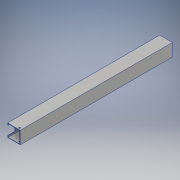
# Autodesk Inventor part: TelescopeOuter
Saved by Autodesk Inventor 2018.3 (Build 223284000, 284)
## iProperties
Created: 2020-01-18
Part Number: TelescopeOuter
Material: Aluminum 6061
Document SubType Name: Modeling
Designer: Cooper
Density: 2.7 g/cm^3
Appearance: Aluminum - Flat
Mass: 387.063 g
Surface Area: 1812.88 cm^2
Volume: 143.357 cm^3
Author: Cooper
Autodesk Inventor part; units mm, degrees
ref_plane "YZ Plane" through (0, 0, 0) normal (1, 0, 0) x (0, 1, 0)
ref_plane "XZ Plane" through (0, 0, 0) normal (0, 1, 0) x (-1, 0, 0)
ref_plane "XY Plane" through (0, 0, 0) normal (0, 0, 1) x (1, 0, 0)
sketch "Sketch1" plane through (0, 0, 0) normal (0, 0, 1) x (1, 0, 0)
  line L0 (0, 0) -> (44.45, 0)
  line L1 (44.45, 0) -> (44.45, 44.45)
  line L2 (44.45, 44.45) -> (0, 44.45)
  line L3 (0, 44.45) -> (0, 0)
  line L4 (1.5875, 42.8625) -> (42.8625, 42.8625)
  line L5 (42.8625, 42.8625) -> (42.8625, 1.5875)
  line L6 (42.8625, 1.5875) -> (1.5875, 1.5875)
  line L7 (1.5875, 1.5875) -> (1.5875, 42.8625)
  dimension "d0" = 44.45
  dimension "d1" = 44.45
  dimension "d2" = 1.5875
  constraints: 16 end point, 4 parallel, 2 perpendicular, 1 horizontal, 3 other
  measures "d0" distance of L2.end L0.start
  measures "d1" distance of L0.start L0.end
  measures "d2" distance between parallel lines of L2 L4
extrude "Extrusion1" add sketch "Sketch1" along normal blind 533.4
sketch "Sketch2" plane through (44.45, 0, 0) normal (1, 0, 0) x (0, 0, -1)
  line L0 (0, 22.225) -> (-12.7, 22.225) construction
  line L1 (0, 12.7) -> (-12.7, 12.7)
  line L2 (-12.7, 31.75) -> (0, 31.75)
  arc A0 (0, 12.7) -> (0, 31.75) centre (0, 22.225) ccw
  arc A1 (-12.7, 31.75) -> (-12.7, 12.7) centre (-12.7, 22.225) ccw
  line L3 (0, 0) -> (0, 44.45) projected
  line L4 (0, 44.45) -> (-533.4, 44.45) projected
  point P0 (-6.35, 22.225)
  dimension "d5" = 0
  dimension "d7" = 19.05
  dimension "d20" = 12.7
  dimension "d21" = 22.225
  constraints: 8 end point, 4 point on circle, 4 tangent, 2 centre point, 1 horizontal, 1 midpoint, 1 parallel, 1 other
  measures "d7" distance between parallel lines of L1 L2
  measures "d20" distance of L1.start L1.end
  measures "d21" distance from line of L4 point (-6.35, 22.225)
extrude "Extrusion2" cut sketch "Sketch2" against normal blind 127
sketch "Sketch6" plane through (44.45, 0, 533.4) normal (1, 0, 0) x (0, 0, -1)
  line L0 (533.4, 42.8625) -> (533.4, 31.75) projected
  arc A0 (520.7, 31.75) -> (520.7, 12.7) centre (520.7, 22.225) ccw projected
  line L1 (533.4, 31.75) -> (520.7, 31.75)
  arc A1 (520.7, 31.75) -> (520.7, 12.7) centre (520.7, 22.225) ccw
  line L2 (533.4, 12.7) -> (520.7, 12.7) projected
  line L3 (520.7, 12.7) -> (533.4, 12.7)
  line L4 (533.4, 12.7) -> (533.4, 31.75)
  point P0 (533.4, 0)
  constraints: 6 end point, 2 horizontal, 2 point on circle, 2 tangent, 1 centre point, 1 perpendicular
extrude "Extrusion3" add sketch "Sketch6" against normal blind 1.5875
sketch "Sketch7" plane through (0, 0, 533.4) normal (-1, 0, 0) x (0, 0, 1)
  line L0 (0, 0) -> (0, 44.45) projected
  line L1 (0, 38.1) -> (-25.4, 38.1)
  line L2 (-25.4, 38.1) -> (-25.4, 6.35)
  line L3 (-25.4, 6.35) -> (0, 6.35)
  line L4 (0, 6.35) -> (0, 38.1)
  line L5 (-39.9502, 6.35) -> (-39.9502, 38.1)
  line L6 (-533.4, 31.75) -> (-520.7, 31.75) projected
  arc A0 (-520.7, 12.7) -> (-520.7, 31.75) centre (-520.7, 22.225) ccw projected
  line L7 (-520.7, 12.7) -> (-533.4, 12.7) projected
  line L8 (-533.4, 12.7) -> (-533.4, 0) projected
  line L9 (-533.4, 0) -> (0, 0) projected
  line L10 (0, 44.45) -> (0, 0) projected
  line L11 (-533.4, 44.45) -> (0, 44.45) projected
  line L12 (-533.4, 44.45) -> (-533.4, 31.75) projected
  dimension "d24" = 25.4
  dimension "d25" = 31.75
  dimension "d26" = 6.35
  dimension "d27" = 6.35
  constraints: 10 end point, 2 parallel, 1 horizontal, 1 perpendicular, 1 point on line, 1 vertical, 2 other
  measures "d24" distance of L1.start L1.end
  measures "d25" distance of L1.end L2.end
  measures "d26" distance between parallel lines of L1 L11
  measures "d27" distance between parallel lines of L9 L3
extrude "Extrusion4" cut sketch "Sketch7" against normal blind 1.5875 contours L3 L2 L1 L0
sketch "Sketch8" plane through (0, 0, 0) normal (0, -1, 0) x (1, 0, 0)
  line L0 (44.45, 0) -> (44.45, 533.4) projected
  line L1 (0, 533.4) -> (44.45, 533.4) projected
  point P0 (0, 0)
  point P1 (35.7188, 527.05)
  dimension "d30" = 8.7312
  dimension "d31" = 6.35
  measures "d30" distance from line of L0 point (35.719, 527.05)
  measures "d31" distance from line of L1 point (35.719, 527.05)
hole "Hole2" at (35.7188, 0, 527.05) direction (0, 1, 0) diameter 5.1562 depth 76.2 tip angle 118
equation "\"d26\" = d27"
body "Solid1"
